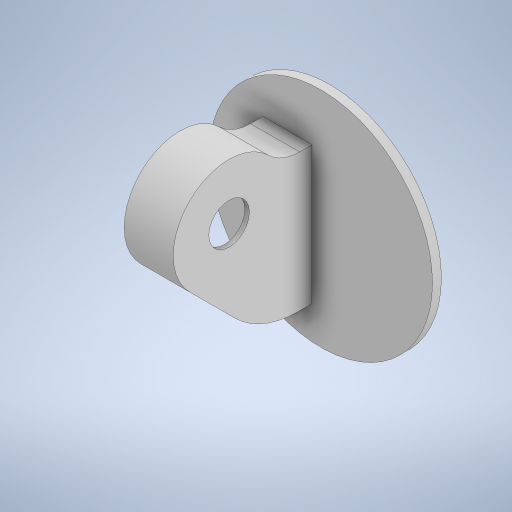
# Autodesk Inventor part: Final Waist
Saved by Autodesk Inventor 2024.1 (Build 281209000, 209)
## iProperties
Created: 2023-12-01
Part Number: Final Waist
Material: Generic
Document SubType Name: Modeling
Designer: vilas
Density: 1 g/cm^3
Appearance: Default
Author: vilas
Autodesk Inventor part; units mm, degrees
ref_plane "XZ Plane" through (0, 0, 0) normal (0, 1, 0) x (-1, 0, 0)
ref_plane "XY Plane" through (0, 0, 0) normal (0, 0, 1) x (1, 0, 0)
sketch "Sketch1" plane through (0, 0, 0) normal (0, 0, 1) x (1, 0, 0)
  circle A0 centre (0, 0) radius 125
  dimension "d0" = 250
  constraints: 1 centre point, 1 coincident
  measures "d0" diameter of A0
extrude "Extrusion1" add sketch "Sketch1" along normal blind 10
ref_plane "Work Plane1" through (-10, 0, 0) normal (1, 0, 0) x (0, 1, 0)
sketch "Sketch2" plane through (-10, 0, 0) normal (1, 0, 0) x (0, 1, 0)
  line L0 (0, 0) -> (0, 156.8689) construction
  line L1 (125, 10) -> (-125, 10) projected
  line L2 (0, 10) -> (-87.5, 10)
  line L3 (-87.5, 10) -> (-87.5, 67.2767)
  line L4 (0, 10) -> (66.5, 10)
  line L5 (66.5, 10) -> (66.5, 44.5)
  line L6 (66.5, 44.5) -> (80.6421, 58.6421)
  line L7 (66.5, 44.5) -> (86.5, 44.5) construction
  line L8 (80.6421, 58.6421) -> (-7.7462, 147.0305) construction
  arc A0 (80.6421, 58.6421) -> (-7.7462, 147.0305) centre (36.448, 102.8363) ccw
  line L9 (-7.7462, 147.0305) -> (-87.5, 67.2767)
  line L10 (-7.7462, 147.0305) -> (127.2538, 147.0305) construction
  circle A1 centre (36.448, 102.8363) radius 22.75
  dimension "d4" = 87.5
  dimension "d6" = 66.5
  dimension "d7" = 34.5
  dimension "d8" = 20
  dimension "d9" = 45
  dimension "d10" = 125
  dimension "d11" = 135
  dimension "d12" = 45.5
  constraints: 20 end point, 2 centre point, 2 horizontal, 2 midpoint, 2 perpendicular, 2 point on circle, 2 point on line, 1 coincident, 1 equal length, 1 vertical
  measures "d4" distance of L2.start L2.end
  measures "d6" distance of L2.start L4.end
  measures "d7" distance of L4.end L5.end
  measures "d8" distance of L5.end L6.end
  measures "d9" angle of L7 L6
  measures "d10" distance of L6.end L8.end
  measures "d11" angle of L9 L10
  measures "d12" diameter of A1
extrude "Extrusion2" add sketch "Sketch2" against normal blind 55
fillet "Fillet1" radius 100 1 edges at (-37.5, -87.5, 67.2767)
fillet "Fillet2" radius 50 1 edges at (-37.5, 66.5, 44.5)
sketch "Sketch3" plane through (-65, 0, 0) normal (-1, 0, 0) x (0, 0, 1)
  line L0 (25.8553, -87.5) -> (10, -87.5) projected
  line L1 (10, -87.5) -> (25.8553, -87.5)
  arc A0 (25.8553, -87.5) -> (96.566, -58.2107) centre (25.8553, 12.5) ccw projected
  arc A1 (25.8553, -87.5) -> (96.566, -58.2107) centre (25.8553, 12.5) ccw
  line L2 (96.566, -58.2107) -> (147.0305, -7.7462) projected
  line L3 (96.566, -58.2107) -> (147.0305, -7.7462)
  arc A2 (147.0305, -7.7462) -> (58.6421, 80.6421) centre (102.8363, 36.448) ccw projected
  arc A3 (147.0305, -7.7462) -> (58.9231, 80.9213) centre (102.8363, 36.448) ccw
  arc A4 (23.7925, 66.5) -> (58.9231, 80.9213) centre (23.7925, 116.5) ccw projected
  arc A5 (23.7925, 66.5) -> (58.9231, 80.9213) centre (23.7925, 116.5) ccw
  line L4 (44.5, 66.5) -> (10, 66.5) projected
  line L5 (23.7925, 66.5) -> (10, 66.5)
  line L6 (10, 66.5) -> (10, -87.5)
  arc A6 (139.9594, -0.6751) -> (65.9492, 73.8056) centre (102.8363, 36.448) ccw
  line L7 (139.9594, -0.6751) -> (117.7788, -23.5781)
  line L8 (0, 0) -> (182.0155, 0) construction
  line L9 (0, -125) -> (0, 125) construction
  line L10 (10, 0) -> (10, -65) construction
  line L11 (10, -65) -> (20, -65)
  arc A7 (20, -65) -> (117.7788, -23.5781) centre (20, 71.1171) ccw
  line L12 (10, 0) -> (10, 40) construction
  arc A8 (10, 40) -> (65.9492, 73.8056) centre (-32.4537, 173.4637) ccw
  dimension "d16" = 10
  dimension "d17" = 65
  dimension "d18" = 10
  dimension "d19" = 40
  constraints: 18 end point, 12 point on circle, 7 tangent, 6 centre point, 4 point on line, 3 collinear, 1 horizontal, 1 perpendicular, 1 vertical
  measures "d16" radial gap between concentric circles of A2 A6
  measures "d17" distance of L10.start L10.end
  measures "d18" distance of L10.end L11.end
  measures "d19" distance of L10.start L12.end
extrude "Extrusion3" cut sketch "Sketch3" against normal blind 19.5 contours L6 A8 A6 L7 A7 L11
sketch "Sketch4" plane through (-45.5, 0, 0) normal (-1, 0, 0) x (0, 0, 1)
  line L0 (143.3452, 39.9686) -> (60.7799, -45.2853) construction
  line L1 (139.9594, -0.6751) -> (117.7788, -23.5781) construction
  circle A0 centre (102.8363, 36.448) radius 22.75 construction
  line L2 (102.2737, 74.1744) -> (28.4952, -2.0066) construction
  line L3 (100.9974, 75.3281) -> (145.8599, 31.8805) construction
  line L4 (22.9611, 6.1258) -> (80.8137, -49.9023) construction
  line L5 (140.5203, 37.0517) -> (68.1686, -37.656)
  line L6 (68.1686, -37.656) -> (29.8809, -0.5758)
  line L7 (29.8809, -0.5758) -> (102.2326, 74.1319)
  line L8 (102.2326, 74.1319) -> (140.5203, 37.0517)
  point P0 (0, 0)
  dimension "d24" = 26.65
  dimension "d25" = 26.65
  dimension "d26" = 26.65
  dimension "d27" = 104
  constraints: 16 end point, 5 parallel, 4 point on line, 2 perpendicular
  measures "d24" distance from line of L2 A0.centre
  measures "d25" distance from line of L0 A0.centre
  measures "d26" distance from line of L3 A0.centre
  measures "d27" distance between parallel lines of L4 L3
extrude "Extrusion4" cut sketch "Sketch4" against normal blind 30.4
sketch "Sketch5" plane through (-45.5, 0, 0) normal (-1, 0, 0) x (0, 0, 1)
  line L0 (147.2746, 42.9) -> (108.2076, 80.7349) construction
  line L1 (102.2326, 74.1319) -> (140.5203, 37.0517) construction
  circle A0 centre (134.4241, 55.3452) radius 3.3
  circle A1 centre (121.0581, 68.2898) radius 3.3
  line L2 (121.3764, 55.5918) -> (127.7411, 61.8175) construction
  line L3 (140.5203, 37.0517) -> (68.1686, -37.656) construction
  line L4 (104.3444, -0.3021) -> (66.0567, 36.7781) construction
  line L5 (29.8809, -0.5758) -> (102.2326, 74.1319) construction
  circle A2 centre (49.6892, -32.149) radius 3.3
  circle A3 centre (36.3231, -19.2044) radius 3.3
  point P0 (0, 0)
  dimension "d30" = 8.9
  dimension "d31" = 6.6
  dimension "d32" = 6.6
  dimension "d33" = 9.3
  dimension "d34" = 9.3
  constraints: 6 end point, 4 centre point, 4 midpoint, 2 point on line, 2 symmetric about line, 1 parallel, 2 other
  measures "d30" distance between parallel lines of L1 L0
  measures "d31" diameter of A0
  measures "d32" diameter of A1
  measures "d33" distance from line of A0.centre L2
  measures "d34" distance from line of A1.centre L2
extrude "Extrusion5" cut sketch "Sketch5" against normal blind 19
body "Solid1"
